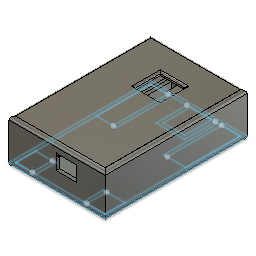
colormeter (Autodesk Fusion 360 design; units mm, degrees)
Autodesk Fusion 360 part; units mm, degrees
sketch "Lolin board" plane through (0, 0, 0) normal (0, 1, 0) x (1, 0, 0) in component "Lolin board"
  line L0 (26, 0) -> (26, 50)
  line L1 (26, 50) -> (0, 50)
  line L2 (15.0596, 6) -> (23.0596, 6)
  circle A0 centre (2.4, 47.6) radius 1
  line L3 (9.5, 8) -> (0, 8)
  circle A1 centre (23.6, 8.5) radius 1
  line L4 (23.0596, 6) -> (23.0596, 0)
  line L5 (15.0596, 0) -> (15.0596, 6)
  line L6 (9.5, 0) -> (9.5, 8)
  line L7 (23.0596, 0) -> (15.0596, 0)
  line L8 (0, 0) -> (26, 0)
  line L9 (0, 0) -> (9.5, 0)
  line L10 (0, 50) -> (0, 0)
  line L11 (0, 8) -> (0, 0)
  point P0 (-10, 5)
  dimension "d5" = 26
  dimension "d6" = 50
  dimension "d7" = 8
  dimension "d8" = 6
  dimension "d9" = 9.5
  dimension "d10" = 8
  dimension "d11" = 2
  dimension "d12" = 2
  constraint horizontal L8
  constraint vertical L0
  constraint horizontal L1
  constraint vertical L10
  constraint horizontal L7
  constraint vertical L5
  constraint horizontal L2
  constraint vertical L4
  constraint coincident L4.end L8
  constraint horizontal L9
  constraint vertical L6
  constraint horizontal L3
  constraint vertical L11
  measures "d5" distance of L8.start L0.start
  measures "d6" distance of L8.start L1.end
  measures "d7" distance of L4.end L5.start
  measures "d8" distance of L4.end L2.end
  measures "d9" distance of L8.start L6.start
  measures "d10" distance of L8.start L3.end
  measures "d11" diameter of A0
  measures "d12" diameter of A1
extrude "Extrude1" add sketch "Lolin board" against normal blind 4.5 makes body 1 in component "Lolin board"
extrude "Extrude2" add sketch "Lolin board" along normal blind 5.7 contours L3 L6 L8 L9 L10 L11 bodies 1 in component "Lolin board"
extrude "Extrude3" add sketch "Lolin board" along normal blind 2.3 contours L2 L4 L5 L7 L8 bodies 1 in component "Lolin board"
sketch "lipo battery" plane through (0, 0, 0) normal (0, 1, 0) x (1, 0, 0) in component "lipo battery"
  line L0 (0, 34) -> (0, 0)
  line L1 (51, 0) -> (51, 34)
  line L2 (51, 34) -> (0, 34)
  line L3 (0, 0) -> (51, 0)
  dimension "d1" = 51
  dimension "d2" = 34
  constraint horizontal L3
  constraint vertical L1
  constraint horizontal L2
  constraint vertical L0
  constraint coincident L0.end L3.start
  measures "d1" distance of L0.end L1.start
  measures "d2" distance of L0.end L0.start
extrude "Extrude1'" add sketch "lipo battery" along normal blind 5.5 separate body makes body 2 in component "lipo battery"
sketch "pcb" plane through (0, 0, 0) normal (0, 1, 0) x (1, 0, 0) in component "colormeter board"
  line L0 (0, 0) -> (30, 0)
  line L1 (30, 0) -> (30, 70)
  line L2 (30, 70) -> (0, 70)
  line L3 (0, 70) -> (0, 0)
  line L4 (24.046, 75.7954) -> (13.546, 75.7954)
  line L5 (13.546, 75.7954) -> (13.546, 61.7954)
  line L6 (13.546, 61.7954) -> (24.046, 61.7954)
  line L7 (24.046, 61.7954) -> (24.046, 75.7954)
  line L8 (21.1116, 60.8091) -> (8.1116, 60.8091)
  line L9 (8.1116, 60.8091) -> (8.1116, 47.8091)
  line L10 (8.1116, 47.8091) -> (21.1116, 47.8091)
  line L11 (21.1116, 47.8091) -> (21.1116, 60.8091)
  dimension "d23" = 30
  dimension "d24" = 70
  dimension "d25" = 10.5
  dimension "d26" = 14
  dimension "d27" = 13
  dimension "d28" = 13
  constraint horizontal L0
  constraint vertical L1
  constraint horizontal L2
  constraint vertical L3
  constraint coincident L0.start L3.end
  constraint horizontal L4
  constraint vertical L5
  constraint horizontal L6
  constraint vertical L7
  constraint horizontal L8
  constraint vertical L9
  constraint horizontal L10
  constraint vertical L11
  measures "d23" distance of L0.start L0.end
  measures "d24" distance of L0.start L2.end
  measures "d25" distance of L4.start L4.end
  measures "d26" distance of L4.start L6.end
  measures "d27" distance of L8.start L8.end
  measures "d28" distance of L8.start L10.end
extrude "Extrude1''" add sketch "pcb" against normal blind 1.5 separate body contours L0 L1 L2 L3 L5 L6 L7 | L2 L5 L6 L7 | L8 L9 L10 L11 makes body 3 in component "colormeter board"
extrude "Extrude2'" add sketch "pcb" against normal blind 9 contours L2 L4 L5 L7 | L2 L5 L6 L7 bodies 3 in component "colormeter board"
extrude "Extrude3'" add sketch "pcb" along normal blind 12 contours L8 L9 L10 L11 bodies 3 in component "colormeter board"
move_body "Move1" bodies 1 to x (1, 0, 0) y (0, 1, 0) z (0, 0, 1) at (2, 4.5, 3) in component "Lolin board"
sketch "Box Bottom" plane through (0, -9, 0) normal (0, -1, 0) x (1, 0, 0) in component "Box Bottom"
  line L0 (24.046, -75.7954) -> (24.046, -61.7954)
  line L1 (24.046, -61.7954) -> (13.546, -61.7954)
  line L2 (13.546, -61.7954) -> (13.546, -75.7954)
  line L3 (13.546, -75.7954) -> (24.046, -75.7954)
  line L4 (42.1029, -76.6879) -> (-11.1899, -76.6879)
  line L5 (-11.1899, -76.6879) -> (-11.1899, 3.9714)
  line L6 (-11.1899, 3.9714) -> (42.1029, 3.9714)
  line L7 (42.1029, 3.9714) -> (42.1029, -76.6879)
  line L8 (-13.1899, -78.6879) -> (-13.1899, 5.9714)
  line L9 (-13.1899, 5.9714) -> (44.1029, 5.9714)
  line L10 (44.1029, 5.9714) -> (44.1029, -78.6879)
  line L11 (44.1029, -78.6879) -> (-13.1899, -78.6879)
  line L12 (28.9871, -44.1619) -> (42.1029, -44.1619)
  line L13 (42.1029, -44.1619) -> (42.1029, -76.6879)
  line L14 (42.1029, -76.6879) -> (28.9871, -76.6879)
  line L15 (28.9871, -76.6879) -> (28.9871, -44.1619)
  line L16 (0.845, -44.1619) -> (-11.1899, -44.1619)
  line L17 (-11.1899, -44.1619) -> (-11.1899, -76.6879)
  line L18 (-11.1899, -76.6879) -> (0.845, -76.6879)
  line L19 (0.845, -76.6879) -> (0.845, -44.1619)
  line L20 (0.845, -7.9317) -> (-11.1899, -7.9317)
  line L21 (-11.1899, -7.9317) -> (-11.1899, 3.9714)
  line L22 (-11.1899, 3.9714) -> (0.845, 3.9714)
  line L23 (0.845, 3.9714) -> (0.845, -7.9317)
  line L24 (29.2087, -7.9317) -> (42.1029, -7.9317)
  line L25 (42.1029, -7.9317) -> (42.1029, 3.9714)
  line L26 (42.1029, 3.9714) -> (29.2087, 3.9714)
  line L27 (29.2087, 3.9714) -> (29.2087, -7.9317)
  line L28 (25.22, -60.4249) -> (12.2569, -60.4249)
  line L29 (12.2569, -60.4249) -> (12.2569, -76.6879)
  line L30 (12.2569, -76.6879) -> (25.22, -76.6879)
  line L31 (25.22, -76.6879) -> (25.22, -60.4249)
  line L32 (27.22, -76.6879) -> (27.22, -58.4249)
  line L33 (27.22, -58.4249) -> (10.2569, -58.4249)
  line L34 (10.2569, -58.4249) -> (10.2569, -76.6879)
  line L35 (-1.155, -76.6879) -> (-1.155, -44.1619)
  line L36 (-1.155, 3.9714) -> (-1.155, -7.9317)
  line L37 (30.9871, -76.6879) -> (30.9871, -44.1619)
  line L38 (31.2087, 3.9714) -> (31.2087, -7.9317)
  dimension "d35" = -2
  dimension "d36" = 2
  dimension "d41" = -2
  dimension "d42" = 2
  dimension "d43" = 2
  dimension "d44" = -2
  constraint horizontal L4
  constraint vertical L5
  constraint horizontal L6
  constraint vertical L7
  constraint horizontal L12
  constraint vertical L13
  constraint horizontal L14
  constraint vertical L15
  constraint horizontal L16
  constraint vertical L17
  constraint horizontal L18
  constraint vertical L19
  constraint horizontal L20
  constraint vertical L21
  constraint horizontal L22
  constraint vertical L23
  constraint horizontal L24
  constraint vertical L25
  constraint horizontal L26
  constraint vertical L27
  constraint horizontal L28
  constraint vertical L29
  constraint horizontal L30
  constraint vertical L31
  constraint coincident L4 L29.end
extrude "Extrude1'''" add sketch "Box Bottom" along normal blind 2 separate body contours L4 L7 L12 L13 L14 L37 | L4 L12 L14 L15 L37 | L4 L5 L6 L7 L12 L15 L16 L19 L20 L23 L24 L27 L32 L33 L34 | L6 L7 L24 L25 L26 L38 | L6 L24 L26 L27 L38 | L6 L20 L22 L23 L36 | L4 L16 L18 L19 L35 | L5 L6 L20 L21 L22 L36 | L4 L5 L16 L17 L18 L35 | L8 L9 L10 L11 makes body 4 in component "Box Bottom"
extrude "Extrude2''" add sketch "Box Bottom" against normal blind 6 contours L4 L7 L12 L13 L14 L37 | L4 L12 L14 L15 L37 | L6 L7 L24 L25 L26 L38 | L6 L24 L26 L27 L38 | L6 L20 L22 L23 L36 | L4 L16 L18 L19 L35 | L5 L6 L20 L21 L22 L36 | L4 L5 L16 L17 L18 L35 | L8 L9 L10 L11 bodies 4 in component "Box Bottom"
extrude "Extrude3''" add sketch "Box Bottom" against normal blind 7.5 contours L4 L7 L12 L13 L14 L37 | L4 L12 L14 L15 L37 | L6 L7 L24 L25 L26 L38 | L6 L24 L26 L27 L38 | L6 L20 L22 L23 L36 | L4 L16 L18 L19 L35 | L5 L6 L20 L21 L22 L36 | L4 L5 L16 L17 L18 L35 bodies 4 in component "Box Bottom"
extrude "Extrude4" add sketch "Box Bottom" against normal blind 9 contours L4 L7 L12 L13 L14 L37 | L6 L7 L24 L25 L26 L38 | L5 L6 L20 L21 L22 L36 | L4 L5 L16 L17 L18 L35 bodies 4 in component "Box Bottom"
extrude "Extrude5" add 1 faces at (43.4362, -3, -38.9595) along direction (0, 1, 0) blind 16 on bodies 4 bodies 4 in component "Box Bottom"
sketch "Box Bottom USB" plane through (0, 0, 5.9714) normal (0, 0, 1) x (1, 0, 0) in component "Box Bottom"
  line L0 (-13.1899, 13) -> (-13.1899, -11)
  line L1 (-13.1899, -11) -> (44.1029, -11)
  line L2 (44.1029, -11) -> (44.1029, 13)
  line L3 (44.1029, 13) -> (-13.1899, 13)
  line L4 (14.9651, 9.9403) -> (26.9651, 9.9403)
  line L5 (26.9651, 9.9403) -> (26.9651, 0.9403)
  line L6 (26.9651, 0.9403) -> (14.9651, 0.9403)
  line L7 (14.9651, 0.9403) -> (14.9651, 9.9403)
  dimension "d51" = 12
  dimension "d52" = 9
  constraint horizontal L4
  constraint vertical L5
  constraint horizontal L6
  constraint vertical L7
  measures "d51" distance of L4.start L4.end
  measures "d52" distance of L4.start L6.end
extrude "Extrude6" cut sketch "Box Bottom USB" against normal blind 3 contours L4 L5 L6 L7 bodies 4 in component "Box Bottom"
sketch "old box top" plane through (0, -9, 0) normal (0, -1, 0) x (1, 0, 0) in component "Box Top"
  line L0 (-13.2324, -78.6592) -> (44.2796, -78.6592)
  line L1 (44.2796, -78.6592) -> (44.2796, 5.9624)
  line L2 (44.2796, 5.9624) -> (-13.2324, 5.9624)
  line L3 (-13.2324, 5.9624) -> (-13.2324, -78.6592)
  line L4 (-11.2324, 3.9624) -> (-11.2324, -76.6592)
  line L5 (-11.2324, -76.6592) -> (42.2796, -76.6592)
  line L6 (42.2796, -76.6592) -> (42.2796, 3.9624)
  line L7 (42.2796, 3.9624) -> (-11.2324, 3.9624)
  line L8 (-11.2324, -31.9033) -> (-9.2324, -31.9033)
  line L9 (-9.2324, -31.9033) -> (-9.2324, -21.9033)
  line L10 (-9.2324, -21.9033) -> (-11.2324, -21.9033)
  line L11 (-11.2324, -21.9033) -> (-11.2324, -31.9033)
  line L12 (42.2796, -31.9196) -> (40.2796, -31.9196)
  line L13 (40.2796, -31.9196) -> (40.2796, -21.9196)
  line L14 (40.2796, -21.9196) -> (42.2796, -21.9196)
  line L15 (42.2796, -21.9196) -> (42.2796, -31.9196)
  line L16 (8.9276, -76.6592) -> (22.9276, -76.6592)
  line L17 (22.9276, -76.6592) -> (22.9276, -74.6592)
  line L18 (22.9276, -74.6592) -> (8.9276, -74.6592)
  line L19 (8.9276, -74.6592) -> (8.9276, -76.6592)
  line L20 (6.9681, -62.0571) -> (21.9542, -62.0571)
  line L21 (21.9542, -62.0571) -> (21.9542, -46.9947)
  line L22 (21.9542, -46.9947) -> (6.9681, -46.9947)
  line L23 (6.9681, -46.9947) -> (6.9681, -62.0571)
  dimension "d55" = -2
  dimension "d56" = 2
  dimension "d57" = 10
  dimension "d58" = 2
  dimension "d59" = 10
  dimension "d60" = 14
  dimension "d61" = 2
  constraint horizontal L0
  constraint vertical L1
  constraint horizontal L2
  constraint vertical L3
  constraint horizontal L8
  constraint vertical L9
  constraint horizontal L10
  constraint vertical L11
  constraint coincident L4 L8.start
  constraint horizontal L12
  constraint vertical L13
  constraint horizontal L14
  constraint vertical L15
  constraint coincident L6 L12.start
  constraint horizontal L16
  constraint vertical L17
  constraint horizontal L18
  constraint vertical L19
  constraint coincident L5 L16.start
  constraint horizontal L20
  constraint vertical L21
  constraint horizontal L22
  constraint vertical L23
  measures "d56" distance of L8.start L8.end
  measures "d57" distance of L8.start L10.end
  measures "d58" distance of L12.start L12.end
  measures "d59" distance of L12.start L14.end
  measures "d60" distance of L16.start L16.end
  measures "d61" distance of L16.start L18.end
sketch "box top" plane through (0, 13, 0) normal (0, 1, 0) x (-1, 0, 0) in component "Box Top"
  line L0 (-42.1029, 3.9714) -> (11.1899, 3.9714)
  line L1 (11.1899, 3.9714) -> (11.1899, -76.6879)
  line L2 (11.1899, -76.6879) -> (-42.1029, -76.6879)
  line L3 (-42.1029, -76.6879) -> (-42.1029, 3.9714)
  line L4 (-44.1029, 5.9714) -> (-44.1029, -78.6879)
  line L5 (-44.1029, -78.6879) -> (13.1899, -78.6879)
  line L6 (13.1899, -78.6879) -> (13.1899, 5.9714)
  line L7 (13.1899, 5.9714) -> (-44.1029, 5.9714)
  line L8 (-8.0724, -74.6592) -> (-22.0724, -74.6592)
  line L9 (-24.0319, -62.0571) -> (-9.0458, -62.0571)
  line L10 (-9.0458, -46.9947) -> (-24.0319, -46.9947)
  line L11 (-42.2324, -21.9033) -> (-42.2324, -31.9033)
  line L12 (-22.0724, -74.6592) -> (-22.0724, -76.6592)
  line L13 (-24.0319, -46.9947) -> (-24.0319, -62.0571)
  line L14 (11.2796, -31.9196) -> (9.2796, -31.9196)
  line L15 (-22.0724, -76.6592) -> (-8.0724, -76.6592)
  line L16 (9.2796, -21.9196) -> (11.2796, -21.9196)
  line L17 (9.2796, -31.9196) -> (9.2796, -21.9196)
  line L18 (11.2796, 3.9624) -> (-42.2324, 3.9624)
  line L19 (13.2796, 5.9624) -> (-44.2324, 5.9624)
  line L20 (-42.2324, 3.9624) -> (-42.2324, -76.6592)
  line L21 (-40.2324, -21.9033) -> (-42.2324, -21.9033)
  line L22 (11.2796, -21.9196) -> (11.2796, -31.9196)
  line L23 (-9.0458, -62.0571) -> (-9.0458, -46.9947)
  line L24 (-8.0724, -76.6592) -> (-8.0724, -74.6592)
  line L25 (-42.2324, -31.9033) -> (-40.2324, -31.9033)
  line L26 (-42.2324, -76.6592) -> (11.2796, -76.6592)
  line L27 (13.2796, -78.6592) -> (13.2796, 5.9624)
  line L28 (-44.2324, 5.9624) -> (-44.2324, -78.6592)
  line L29 (11.2796, -76.6592) -> (11.2796, 3.9624)
  line L30 (-44.2324, -78.6592) -> (13.2796, -78.6592)
  line L31 (-40.2324, -31.9033) -> (-40.2324, -21.9033)
  line L32 (-9.6047, 3.9714) -> (-23.6047, 3.9714)
  line L33 (-23.6047, 3.9714) -> (-23.6047, 1.9714)
  line L34 (-23.6047, 1.9714) -> (-9.6047, 1.9714)
  line L35 (-9.6047, 1.9714) -> (-9.6047, 3.9714)
  point P0 (-31, 0)
  dimension "d62" = -2
  dimension "d63" = 2
  dimension "d64" = 10
  dimension "d65" = 2
  dimension "d66" = 10
  dimension "d67" = 14
  dimension "d68" = 2
  dimension "d75" = 14
  dimension "d76" = 2
  constraint horizontal L30
  constraint vertical L27
  constraint horizontal L19
  constraint vertical L28
  constraint horizontal L25
  constraint vertical L31
  constraint horizontal L21
  constraint vertical L11
  constraint coincident L11.end L20
  constraint horizontal L14
  constraint vertical L17
  constraint horizontal L16
  constraint vertical L22
  constraint coincident L14.start L29
  constraint horizontal L15
  constraint vertical L24
  constraint horizontal L8
  constraint vertical L12
  constraint coincident L12.end L26
  constraint horizontal L9
  constraint vertical L23
  constraint horizontal L10
  constraint vertical L13
  constraint horizontal L32
  constraint vertical L33
  constraint horizontal L34
  constraint vertical L35
  constraint coincident L0 L32.start
  measures "d63" distance of L25.end L11.end
  measures "d64" distance of L11.start L11.end
  measures "d65" distance of L14.end L14.start
  measures "d66" distance of L14.start L16.end
  measures "d67" distance of L12.end L15.end
  measures "d68" distance of L8.end L12.end
  measures "d75" distance of L32.start L32.end
  measures "d76" distance of L32.start L34.end
extrude "Extrude1''''" add sketch "box top" along normal blind 2 separate body contours L1 L3 L8 L12 L14 L16 L17 L18 L21 L24 L25 L26 L31 L33 L34 L35 | L18 L33 L34 L35 | L3 L21 L25 L31 | L1 L14 L16 L17 | L8 L12 L15 L24 L26 | L4 L6 L19 L30 makes body 5 in component "Box Top"
extrude "Extrude2'''" add sketch "box top" against normal blind 2 contours L3 L21 L25 L31 | L1 L14 L16 L17 bodies 5 in component "Box Top"
extrude "Extrude4'" add sketch "box top" against normal blind 13 separate body contours L8 L12 L15 L24 L26 makes body 6 in component "Box Top"
extrude "Extrude3'''" add sketch "box top" against normal blind 6 separate body contours L18 L33 L34 L35 makes body 7 in component "Box Top"
cylinder "CylinderPrimitive1" add diameter 2 height -14 placed x (0, 0, -1) y (0, 1, 0) z (1, 0, 0) at (22.0724, 0.9611, -76.6592) separate body makes body 8 in component "Box Top"
cylinder "CylinderPrimitive2" add diameter 2 height -14 placed x (0, 0, -1) y (0, 1, 0) z (1, 0, 0) at (23.6047, 8.0044, 3.9624) separate body makes body 9 in component "Box Top"
combine "Combine1" operation cut target body 4 tool bodies 8 9 keep tools in component "Box Bottom"
move_face "OffsetFaces1" offset -0.5 1 faces at (14.2714, 9, 3.9624) on bodies 7 in component "Box Top"
move_face "OffsetFaces2" offset -0.5 1 faces at (17.4057, 8.6667, -76.6592) on bodies 6 in component "Box Top"
move_body "Move1'" bodies 8 to x (1, 0, 0) y (0, 1, 0) z (0, 0, 1) at (0, 0, 0.5) in component "Box Top"
move_body "Move2" bodies 9 to x (1, 0, 0) y (0, 1, 0) z (0, 0, 1) at (0, 0, -0.5) in component "Box Top"
combine "Combine1'" operation add target body 5 tool bodies 6 7 8 9 in component "Box Top"
fillet "Fillet1" radius 1 4 edges at (9.0458, 15, -54.5259) (16.5389, 15, -62.0571) (24.0319, 15, -54.5259) (16.5389, 15, -46.9947) on bodies 5 in component "Box Top"
fillet "Fillet2" radius 2 4 edges at (15.4565, 15, 5.9624) (-13.1899, 15, -36.3484) (15.4565, 15, -78.6592) (44.1029, 15, -36.3484) on bodies 5 in component "Box Top"
fillet "Fillet1'" radius 2 4 edges at (44.1029, -11, -36.3582) (15.4565, -11, 5.9714) (-13.1899, -11, -36.3582) (15.4565, -11, -78.6879) on bodies 4 in component "Box Bottom"
box "BoxPrimitive1" add length 2 width 14 height 8 placed x (0, 1, 0) y (-1, 0, 0) z (0, 0, 1) at (22.0724, 0, -74.6592) separate body makes body 10 in component "Box Top"
fillet "Fillet3" radius 1 2 edges at (15.0724, 0, -66.6592) (15.0724, 2, -66.6592) on bodies 10 in component "Box Top"
combine "Combine2" operation add target body 5 tool bodies 10 in component "Box Top"
fillet "Fillet4" radius 1 1 edges at (15.0724, 2, -74.6592) on bodies 5 in component "Box Top"
extrude "Extrude5'" cut sketch "Box Bottom USB" against normal blind 4 contours L4 L5 L6 L7 bodies 5 in component "Box Top"
component "colormeter board" placed x (1, 0, 0) y (0, 1, 0) z (0, 0, 1) at (0, 0, 0)
component "Box Bottom" placed x (1, 0, 0) y (0, 1, 0) z (0, 0, 1) at (0, 0, 0)
component "Box Top" placed x (1, 0, 0) y (0, 1, 0) z (0, 0, 1) at (0, 0, 0)
component "Lolin board" placed x (1, 0, 0) y (0, 1, 0) z (0, 0, 1) at (0, 0, 0) in component "colormeter board"
component "lipo battery" placed x (1, 0, 0) y (0, 1, 0) z (0, 0, 1) at (-10, 6, -9) in component "colormeter board"
named bodies: "lipo battery", "Lolin board", "pcb", "Box Bottom", "Box Top"
